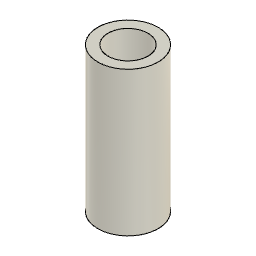
Strain_Relief_Spacer_36STH20 (Autodesk Fusion 360 design; units mm, degrees)
Autodesk Fusion 360 part; units mm, degrees
sketch "Sketch1" plane through (0, 0, 0) normal (0, 0, 1) x (1, 0, 0)
  circle A0 centre (0, 0) radius 3.55
  dimension "d1" = 7.1
  constraint coincident A0.centre origin
  measures "d1" diameter of A0
extrude "Extrude1" add sketch "Sketch1" along normal blind 17
hole "Hole1" at (0, 0, 17) direction (0, 0, -1) diameter 4.7 depth 5 tip angle 180
hole "Hole2" at (0, 0, 0) direction (0, 0, 1) diameter 4.7 depth 5 tip angle 180
